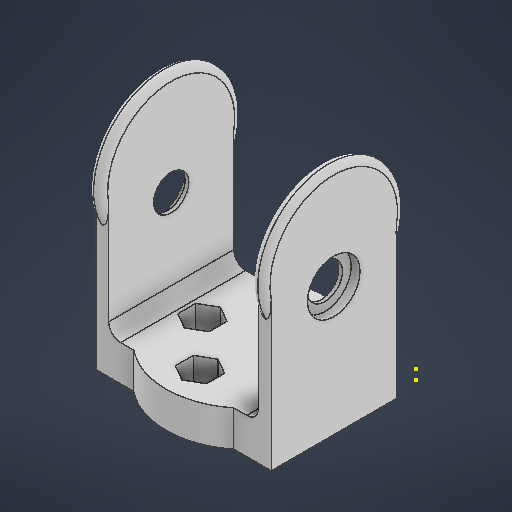
# Autodesk Inventor part: Robot_piece
Saved by Autodesk Inventor 2026.1 (Build 301233000, 233)
## iProperties
Created: 2025-07-26
Part Number: Robot_piece
Material: Generic
Document SubType Name: Modeling
Designer: Fffar
Density: 1 g/cm^3
Appearance: Default
Author: Fffar
Autodesk Inventor part; units mm, degrees
ref_plane "YZ Plane" through (0, 0, 0) normal (1, 0, 0) x (0, 1, 0)
ref_plane "XZ Plane" through (0, 0, 0) normal (0, 1, 0) x (-1, 0, 0)
ref_plane "XY Plane" through (0, 0, 0) normal (0, 0, 1) x (1, 0, 0)
sketch "Sketch1" plane through (0, 0, 0) normal (0, 0, 1) x (1, 0, 0)
  line L0 (-70.0569, -9.2274) -> (-65.5569, -9.2274)
  line L1 (-65.5569, -9.2274) -> (-65.5569, 48.7726)
  line L2 (-65.5569, 48.7726) -> (-70.0569, 48.7726)
  line L3 (-70.0569, 48.7726) -> (-70.0569, -9.2274)
  line L4 (-11.5569, -9.2274) -> (-7.0569, -9.2274)
  line L5 (-7.0569, -9.2274) -> (-7.0569, 48.7726)
  line L6 (-7.0569, 48.7726) -> (-11.5569, 48.7726)
  line L7 (-11.5569, 48.7726) -> (-11.5569, -9.2274)
  line L8 (-65.5569, 3.626) -> (-11.5569, 3.626)
  line L9 (-11.5569, 3.626) -> (-11.5569, -9.2274)
  line L10 (-11.5569, -9.2274) -> (-65.5569, -9.2274)
  line L11 (-65.5569, -9.2274) -> (-65.5569, 3.626)
  point P0 (0, 0)
  point P1 (-11.5569, 3.626)
  dimension "d5" = 4.5
  dimension "d6" = 58
  dimension "d8" = 4.5
  dimension "d9" = 58
  dimension "d10" = 54
  constraints: 24 end point, 6 parallel, 3 horizontal, 3 perpendicular, 1 point on line
  measures "d5" distance of L1.end L2.end
  measures "d6" distance of L2.end L0.start
  measures "d8" distance of L5.end L6.end
  measures "d9" distance of L6.end L4.start
  measures "d10" distance of L8.start L8.end
sketch "Sketch2" plane through (0, 0, 0) normal (0, 0, 1) x (1, 0, 0)
  point P0 (0, 0)
sketch "Sketch3" plane through (0, 0, 0) normal (0, 0, 1) x (1, 0, 0)
  point P0 (0, 0)
sketch "Sketch4" plane through (0, 0, 0) normal (1, 0, 0) x (0, 1, 0)
  point P0 (0, 0)
sketch "Sketch5" plane through (0, 0, 0) normal (0, 0, 1) x (1, 0, 0)
  point P0 (0, 0)
sketch "Sketch6" plane through (0, 0, 0) normal (0, 0, 1) x (1, 0, 0)
  point P0 (0, 0)
extrude "Extrusion1" add sketch "Sketch1" along normal blind 45
sketch "Sketch7" plane through (-65.5569, 3.626, 0) normal (0, 1, 0) x (1, 0, 0)
  line L0 (54, 0) -> (0, 0) projected
  circle A0 centre (27, -22.5044) radius 28.8047
  line L1 (54, 0) -> (54, -45) projected
  circle A1 centre (27, -8.5344) radius 4.0997
  line L2 (54, -45) -> (0, -45) projected
  line L3 (0, 0) -> (0, -45) projected
  circle A2 centre (27.071, -36.4744) radius 4.0997
  circle A3 centre (11.76, -22.5044) radius 4.0997
  circle A4 centre (42.9256, -22.5044) radius 4.0997
  point P0 (65.5569, 0)
  point P1 (0, -22.5)
  point P2 (54, -22.5)
  point P3 (0, -12.4688)
  point P4 (0, -32.54)
  point P5 (54, -32.54)
  point P6 (54, -12.4688)
  dimension "d16" = 22.5044
  dimension "d17" = 27
  dimension "d18" = 27
  dimension "d19" = 13.97
  dimension "d20" = 22.4956
  dimension "d21" = 27
  dimension "d22" = 13.97
  dimension "d23" = 0
  dimension "d24" = 15.24
  dimension "d25" = 11.0744
  dimension "d26" = 0
  constraints: 5 centre point, 2 midpoint
  measures "d16" distance from line of L0 A0.centre
  measures "d17" distance from line of L1 A0.centre
  measures "d18" distance from line of L1 A1.centre
  measures "d19" distance of A0.centre A1.centre
  measures "d20" distance from line of L2 A0.centre
  measures "d21" distance of point (0, -22.5) A0.centre
  measures "d22" vertical distance of A0.centre A2.centre
  measures "d23" vertical distance of A0.centre A3.centre
  measures "d24" distance of A0.centre A3.centre
  measures "d25" distance of point (54, -22.5) A4.centre
  measures "d26" vertical distance of A0.centre A4.centre
fillet "Fillet1" radius 4.318 1 edges at (-65.5569, 3.626, 22.5)
fillet "Fillet2" radius 4.318 1 edges at (-11.5569, 3.626, 22.5)
extrude "Extrusion2" add sketch "Sketch7" against normal up to surface (12.8534 mm away) contours A0 L1 L2 L3 L0 | L0 A0 | A0 L2
sketch "Sketch9" plane through (-61.2389, 3.626, 45) normal (0, 1, 0) x (1, 0, 0)
  arc A0 (4.6914, 0) -> (40.6726, 0) centre (22.682, 22.4956) ccw projected
  arc A1 (40.6616, 45) -> (4.7024, 45) centre (22.682, 22.4956) ccw projected
  line L0 (-8.818, 45) -> (-8.818, 0) projected
  line L1 (54.182, 0) -> (54.182, 45) projected
  line L2 (22.682, 51.3003) -> (22.682, -6.3091)
  line L3 (22.682, 32.6556) -> (17.0686, 35.8965)
  line L4 (17.0686, 35.8965) -> (17.0686, 42.3784)
  line L5 (17.0686, 42.3784) -> (22.682, 45.6193)
  line L6 (22.682, 45.6193) -> (28.2954, 42.3784)
  line L7 (28.2954, 42.3784) -> (28.2954, 35.8965)
  line L8 (28.2954, 35.8965) -> (22.682, 32.6556)
  line L9 (-8.818, 22.5) -> (54.182, 22.5)
  line L10 (54.182, 45) -> (54.182, 0) projected
  line L11 (22.682, -0.6237) -> (17.0686, 2.6172)
  line L12 (17.0686, 2.6172) -> (17.0686, 9.0991)
  line L13 (17.0686, 9.0991) -> (22.682, 12.34)
  line L14 (22.682, 12.34) -> (28.2954, 9.0991)
  line L15 (28.2954, 9.0991) -> (28.2954, 2.6172)
  line L16 (28.2954, 2.6172) -> (22.682, -0.6237)
  line L17 (38.4554, 15.9599) -> (32.842, 19.2008)
  line L18 (32.842, 19.2008) -> (32.842, 25.6826)
  line L19 (32.842, 25.6826) -> (38.4554, 28.9236)
  line L20 (38.4554, 28.9236) -> (44.0689, 25.6826)
  line L21 (44.0689, 25.6826) -> (44.0689, 19.2008)
  line L22 (44.0689, 19.2008) -> (38.4554, 15.9599)
  line L23 (6.9086, 16.0182) -> (1.2951, 19.2591)
  line L24 (1.2951, 19.2591) -> (1.2951, 25.7409)
  line L25 (1.2951, 25.7409) -> (6.9086, 28.9818)
  line L26 (6.9086, 28.9818) -> (12.522, 25.7409)
  line L27 (12.522, 25.7409) -> (12.522, 19.2591)
  line L28 (12.522, 19.2591) -> (6.9086, 16.0182)
  point P0 (61.2389, 45)
  point P1 (22.682, 39.1374)
  point P2 (22.682, 22.4956)
  point P3 (22.682, 5.8582)
  point P4 (22.682, 22.5)
  point P5 (38.4554, 22.4417)
  point P6 (32.842, 22.4417)
  point P7 (6.9086, 22.5)
  point P8 (12.522, 22.5)
  dimension "d49" = 57.6095
  dimension "d50" = 63
  dimension "d51" = 10.16
  dimension "d52" = 10.16
  dimension "d53" = 0
  dimension "d54" = 10.16
  dimension "d55" = 10.16
  dimension "d56" = 0
  constraints: 52 end point, 6 midpoint, 2 point on circle, 2 point on line, 1 perpendicular, 1 vertical, 52 other
  measures "d49" distance of L2.end L2.start
  measures "d50" distance of L9.start L9.end
  measures "d51" distance of L3.start point (22.682, 22.496)
  measures "d52" distance of point (22.682, 22.5) L13.end
  measures "d53" distance from line of L2 point (22.682, 5.858)
  measures "d54" horizontal distance of A0.centre point (32.842, 22.442)
  measures "d55" distance of point (22.682, 22.496) point (12.522, 22.5)
  measures "d56" distance from line of L9 point (6.909, 22.5)
sketch "Sketch10" plane through (-61.2389, 3.626, 45) normal (0, 1, 0) x (1, 0, 0)
  point P0 (61.2389, 45)
extrude "Extrusion4" cut sketch "Sketch9" against normal up to surface (12.8534 mm away)
sketch "Sketch11" plane through (-7.0569, -9.2274, 0) normal (1, 0, 0) x (0, 0, -1)
  line L0 (-45, 0) -> (-45, 58) projected
  line L1 (0, 0) -> (0, 58) projected
  line L2 (0, 58) -> (-45, 58) projected
  line L3 (0, 0) -> (-45, 0) projected
  line L4 (-22.5, 0) -> (-22.5, 58)
  line L5 (0, 46.7868) -> (-45, 46.7868)
  circle A0 centre (-22.5, 58) radius 25.4
  line L6 (-22.5, 58) -> (-22.5, 0)
  point P0 (0, 9.2274)
  point P1 (-45, 46.214)
  point P2 (0, 46.214)
  dimension "d59" = 45
  dimension "d60" = 58
  dimension "d61" = 46.7868
  dimension "d62" = 50.8
  constraints: 6 end point, 2 midpoint, 2 perpendicular, 2 point on line, 1 centre point, 1 coincident, 1 vertical
  measures "d59" distance between parallel lines of L0 L1
  measures "d60" distance of L4.end L4.start
  measures "d61" distance of L1.start L5.start
  measures "d62" diameter of A0
extrude "Extrusion5" add sketch "Sketch11" against normal up to surface (4.5 mm away) contours L0 A0 L1 L2
sketch "Sketch12" plane through (-70.0569, -9.2274, 0) normal (-1, 0, 0) x (0, 0, 1)
  line L0 (25.7992, 0) -> (19.3174, 0) projected
  line L1 (22.5583, 0) -> (22.5, 58)
  line L2 (0, 58) -> (45, 58) projected
  circle A0 centre (22.5, 58) radius 25.4
  point P0 (0, 9.2274)
  dimension "d65" = 50.8
  constraints: 2 end point, 2 midpoint, 1 centre point, 1 coincident
  measures "d65" diameter of A0
extrude "Extrusion6" add sketch "Sketch12" against normal up to surface (4.5 mm away)
sketch "Sketch13" plane through (-70.0569, -9.2274, 0) normal (-1, 0, 0) x (0, 0, 1)
  line L0 (0, 0) -> (45, 0) projected
  arc A0 (45, 46.214) -> (0, 46.214) centre (22.5, 58) ccw projected
  line L1 (0, 17.1714) -> (0, 46.214) projected
  line L2 (0, 46.214) -> (45, 46.214)
  line L3 (22.5, 83.4) -> (22.5, 0)
  line L4 (25.7992, 12.8534) -> (25.7992, 0) projected
  circle A1 centre (22.5, 46.214) radius 9.4673
  circle A2 centre (22.5, 46.214) radius 9.4673
  point P0 (0, 9.2274)
  dimension "d68" = 83.4
  constraints: 4 end point, 2 centre point, 2 midpoint, 1 coincident, 1 parallel, 1 perpendicular, 1 point on circle, 1 point on line
  measures "d68" distance of L3.end L3.start
extrude "Extrusion7" cut sketch "Sketch13" against normal blind 3.175 contours A1 L3 L2 | L2 L3 A1 | L3 L2 A1 | L3 A1 L2
sketch "Sketch14" plane through (-7.0569, -9.2274, 45) normal (1, 0, 0) x (0, 0, -1)
  circle A0 centre (22.5, 46.214) radius 9.4673 projected
  circle A1 centre (22.5, 46.214) radius 9.4673
  point P0 (45, 9.2274)
  constraints: 1 centre point, 1 coincident
extrude "Extrusion8" cut sketch "Sketch14" against normal blind 3.175
sketch "Sketch15" plane through (-10.2319, 36.9866, 22.5) normal (1, 0, 0) x (0, 0, -1)
  circle A0 centre (0, 0) radius 6.35
  circle A1 centre (0, 0) radius 6.35
  circle A2 centre (0, 0) radius 6.35
  point P0 (22.5, -36.9866)
  dimension "d73" = 12.7
  dimension "d74" = 12.7
  constraints: 3 centre point, 2 coincident, 1 concentric
  measures "d73" diameter of A0
  measures "d74" diameter of A1
extrude "Extrusion9" cut sketch "Sketch15" against normal blind 3.175
sketch "Sketch16" plane through (-66.8819, 36.9866, 22.5) normal (-1, 0, 0) x (0, 0, 1)
  circle A0 centre (0, 0) radius 6.35 projected
  circle A1 centre (0, 0) radius 6.35
  point P0 (-22.5, -36.9866)
  constraints: 1 centre point, 1 coincident
extrude "Extrusion10" cut sketch "Sketch16" against normal blind 3.175
fillet "Fillet7" radius 2.54 1 edges at (-11.5569, 74.1726, 22.5)
fillet "Fillet8" radius 2.54 1 edges at (-65.5569, 74.1726, 22.5)
fillet "Fillet9" radius 2.54 1 edges at (-7.0569, 74.1726, 22.5)
fillet "Fillet10" radius 2.54 1 edges at (-70.0569, 74.1726, 22.5)
body "Solid1"
